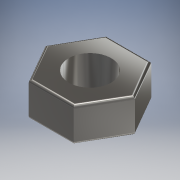
# Autodesk Inventor part: m3 nut
Saved by Autodesk Inventor 2017 (Build 210142000, 142)
## iProperties
Created: 2019-12-06
Part Number: m3 nut
Material: Generic
Document SubType Name: Modeling
Designer: User
Density: 1 g/cm^3
Appearance: Default
Mass: 0.0455871 g
Surface Area: 1.03293 cm^2
Volume: 0.0455871 cm^3
Author: User
Autodesk Inventor part; units mm, degrees
ref_plane "YZ Plane" through (0, 0, 0) normal (1, 0, 0) x (0, 1, 0)
ref_plane "XZ Plane" through (0, 0, 0) normal (0, 1, 0) x (-1, 0, 0)
ref_plane "XY Plane" through (0, 0, 0) normal (0, 0, 1) x (1, 0, 0)
sketch "Sketch1" plane through (0, 0, 0) normal (0, 0, 1) x (1, 0, 0)
  circle A0 centre (0, 0) radius 1.5
  line L0 (-1.5877, 2.75) -> (1.5877, 2.75)
  line L1 (1.5877, -2.75) -> (-1.5877, -2.75)
  line L2 (1.5877, 2.75) -> (3.1754, 0)
  line L3 (3.1754, 0) -> (1.5877, -2.75)
  line L4 (-1.5877, 2.75) -> (-3.1754, 0)
  line L5 (-3.1754, 0) -> (-1.5877, -2.75)
  dimension "d0" = 3
  constraints: 12 end point, 1 centre point, 1 coincident, 1 horizontal, 1 parallel
  measures "d0" diameter of A0
extrude "Extrusion1" add sketch "Sketch1" along normal blind 2.4
fillet "Fillet1" radius 0.2 12 edges at (0, 2.75, 2.4) (2.3816, 1.375, 2.4) (2.3816, -1.375, 2.4) (0, -2.75, 2.4) (-2.3816, -1.375, 2.4) (-2.3816, 1.375, 2.4) (0, 2.75, 0) (2.3816, 1.375, 0) (2.3816, -1.375, 0) (-2.3816, -1.375, 0) (0, -2.75, 0) (-2.3816, 1.375, 0)
body "Solid1"
